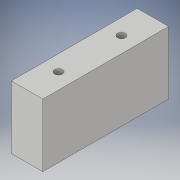
# Autodesk Inventor part: Slider
Saved by Autodesk Inventor 2019 (Build 230136000, 136)
## iProperties
Created: 2019-09-28
Part Number: Slider
Material: Generic
Document SubType Name: Modeling
Designer: james
Density: 1 g/cm^3
Appearance: Default
Author: james
Autodesk Inventor part; units mm, degrees
ref_plane "YZ Plane" through (0, 0, 0) normal (1, 0, 0) x (0, 1, 0)
ref_plane "XZ Plane" through (0, 0, 0) normal (0, 1, 0) x (-1, 0, 0)
ref_plane "XY Plane" through (0, 0, 0) normal (0, 0, 1) x (1, 0, 0)
sketch "Sketch1" plane through (0, 0, 0) normal (0, 0, 1) x (1, 0, 0)
  line L0 (-12.552, 15.5925) -> (0.148, 15.5925)
  line L1 (0.148, 15.5925) -> (0.148, -9.8075)
  line L2 (0.148, -9.8075) -> (-12.552, -9.8075)
  line L3 (-12.552, -9.8075) -> (-12.552, 15.5925)
  point P0 (0, 0)
  dimension "d0" = 12.7
  dimension "d1" = 25.4
  constraints: 8 end point, 2 parallel, 1 horizontal, 1 perpendicular
  measures "d0" distance of L1.end L2.end
  measures "d1" distance of L2.end L0.start
extrude "Extrusion1" add sketch "Sketch1" along normal blind 50.8
sketch "Sketch2" plane through (-12.552, 15.5925, 0) normal (0, 1, 0) x (1, 0, 0)
  line L0 (12.7, -50.8) -> (0, -50.8) projected
  line L1 (12.7, 0) -> (12.7, -50.8) projected
  point P0 (12.552, 0)
  point P1 (6.35, -38.1)
  point P2 (6.35, -12.7)
  dimension "d4" = 25.4
  dimension "d5" = 12.7
  dimension "d6" = 0
  dimension "d7" = 6.35
  measures "d4" distance of point (6.35, -38.1) point (6.35, -12.7)
  measures "d5" distance from line of L0 point (6.35, -38.1)
  measures "d6" horizontal distance of point (6.35, -38.1) point (6.35, -12.7)
  measures "d7" distance from line of L1 point (6.35, -12.7)
hole "Hole1" at (-6.202, 15.5925, 38.1) at (-6.202, 15.5925, 12.7) direction (0, -1, 0) diameter 3.175 end through all
body "Solid1"
